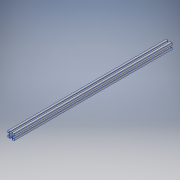
# Autodesk Inventor part: 20x20 Extrusion with threaded end
Saved by Autodesk Inventor 2020.2 (Build 242310000, 310)
## iProperties
Created: 2018-06-16
Part Number: 20x20 Extrusion with threaded end
Material: Aluminum 6061
Document SubType Name: Modeling
Designer: Richard
Density: 2.7 g/cm^3
Appearance: Aluminum - Flat
Author: Richard
Autodesk Inventor part; units mm, degrees
ref_plane "YZ Plane" through (0, 0, 0) normal (1, 0, 0) x (0, 1, 0)
ref_plane "XZ Plane" through (0, 0, 0) normal (0, 1, 0) x (-1, 0, 0)
ref_plane "XY Plane" through (0, 0, 0) normal (0, 0, 1) x (1, 0, 0)
sketch "Sketch1" plane through (0, 0, 0) normal (0, 0, 1) x (1, 0, 0)
  line L0 (-10, -10) -> (10, -10)
  line L1 (10, -10) -> (10, 10)
  line L2 (10, 10) -> (-10, 10)
  line L3 (-10, 10) -> (-10, -10)
  line L4 (-10, -10) -> (10, 10) construction
  line L5 (10, -10) -> (-10, 10) construction
  point P0 (0, 0)
  dimension "d0" = 20
  dimension "d1" = 20
  constraints: 12 end point, 2 collinear, 2 midpoint, 1 perpendicular, 1 vertical
  measures "d0" distance of L2.end L1.end
  measures "d1" distance of L1.end L0.end
extrude "Extrusion1" add sketch "Sketch1" along normal mid plane 500
sketch "Sketch2" plane through (0, 0, 250) normal (0, 0, 1) x (1, 0, 0)
  line L0 (-10, -10) -> (10, -10) projected
  line L1 (10, -10) -> (10, 10) projected
  line L2 (10, 10) -> (-10, 10) projected
  line L3 (-10, 10) -> (-10, -10) projected
  line L4 (10, 10) -> (-10, 10) projected
  line L5 (-3, 10) -> (-3, 8)
  line L6 (-3, 8) -> (-6, 8)
  line L7 (-3, 4) -> (3, 4)
  line L8 (6, 8) -> (3, 8)
  line L9 (3, 8) -> (3, 10)
  line L10 (-3, 4) -> (-6, 7)
  line L11 (-6, 7) -> (-6, 8)
  line L12 (3, 4) -> (6, 7)
  line L13 (6, 7) -> (6, 8)
  line L14 (-0.35, 4) -> (0, 3.75)
  line L15 (0, 3.75) -> (0.35, 4)
  point P0 (0, 0)
  point P1 (0, 4)
  dimension "d5" = 2
  dimension "d6" = 4
  dimension "d7" = 12
  dimension "d8" = 6
  dimension "d9" = 1
  dimension "d10" = 6
  dimension "d11" = 6
  dimension "d25" = 0.25
  dimension "d26" = 0.7
  constraints: 22 end point, 6 point on line, 3 equal length, 3 perpendicular, 2 parallel, 2 vertical alignment, 1 midpoint, 1 vertical
  measures "d5" distance of L5.start L5.end
  measures "d6" distance between parallel lines of L6 L7
  measures "d7" distance between parallel lines of L13 L11
  measures "d8" distance between parallel lines of L9 L5
  measures "d9" distance of L10.end L6.end
  measures "d10" distance from line of point (0, 0) L11
  measures "d11" distance of L7.start L7.end
  measures "d25" distance from line of L7 L14.end
  measures "d26" distance of L15.end L14.start
extrude "Extrusion2" cut sketch "Sketch2" against normal through all contours L2 L9 L8 L13 L12 L7 L10 L11 L6 L5 | L7 L15 L14
pattern_circular "Circular Pattern1" count 4 over 360 about axis through (0, 0, -10) along (0, 0, 1) of "Extrusion2"
fillet "Fillet1" radius 1 4 edges at (10, 10, 0) (10, -10, 0) (-10, 10, 0) (-10, -10, 0)
sketch "Sketch6" plane through (0, 0, 250) normal (0, 0, 1) x (1, 0, 0)
  point P0 (0, 0)
  point P1 (0, 0)
  constraints: 1 coincident
hole "Hole3" at (0, 0, 250) direction (0, 0, -1) diameter 4.1 end through all
body "Solid1"
